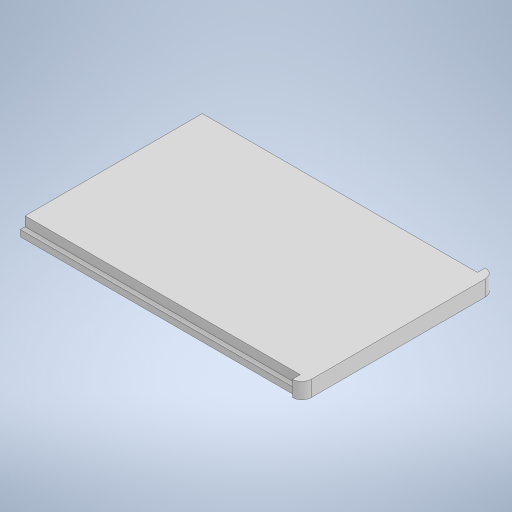
# Autodesk Inventor part: bt-lid
Saved by Autodesk Inventor 2024.2 (Build 282272000, 272)
## iProperties
Created: 2025-05-11
Part Number: bt-lid
Material: Типовые
Document SubType Name: Modeling
Designer: nikit
Density: 1 g/cm^3
Appearance: По умолчанию
Author: nikit
Autodesk Inventor part; units mm, degrees
ref_plane "YZ Plane" through (0, 0, 0) normal (1, 0, 0) x (0, 1, 0)
ref_plane "XZ Plane" through (0, 0, 0) normal (0, 1, 0) x (-1, 0, 0)
ref_plane "XY Plane" through (0, 0, 0) normal (0, 0, 1) x (1, 0, 0)
sketch "Эскиз1" plane through (0, 0, 0) normal (0, 1, 0) x (-1, 0, 0)
  line L0 (43.5, -29.5) -> (-43.5, -29.5)
  line L1 (-43.5, -29.5) -> (-43.5, 29.5)
  line L2 (-43.5, 29.5) -> (43.5, 29.5)
  line L3 (43.5, 29.5) -> (43.5, -29.5)
  line L4 (43.5, -29.5) -> (-43.5, 29.5) construction
  line L5 (-43.5, -29.5) -> (43.5, 29.5) construction
  point P0 (0, 0)
  dimension "d0" = 87
  dimension "d1" = 59
  constraints: 12 end point, 2 midpoint, 2 parallel, 1 horizontal, 1 perpendicular
  measures "d0" distance of L1.end L2.end
  measures "d1" distance of L0.end L1.end
extrude "Выдавливание1" add sketch "Эскиз1" along normal blind 2
sketch "Эскиз2" plane through (0, 2, 0) normal (0, 1, 0) x (1, 0, 0)
  line L0 (43.5, -28) -> (-43.5, -28)
  line L1 (-43.5, -28) -> (-43.5, 28)
  line L2 (-43.5, 28) -> (43.5, 28)
  line L3 (43.5, 28) -> (43.5, -28)
  line L4 (43.5, -28) -> (-43.5, 28) construction
  line L5 (-43.5, -28) -> (43.5, 28) construction
  point P0 (0, 0)
  dimension "d4" = 87
  dimension "d5" = 56
  constraints: 12 end point, 2 midpoint, 2 parallel, 1 horizontal, 1 perpendicular
  measures "d4" distance of L1.end L2.end
  measures "d5" distance of L0.end L1.end
extrude "Выдавливание2" add sketch "Эскиз2" along normal blind 3
sketch "Эскиз3" plane through (0, 0, 0) normal (0, -1, 0) x (1, 0, 0)
  line L0 (43.5, 29.5) -> (43.5, -29.5) projected
  line L1 (43.5, 0) -> (43.5, -30.5)
  line L2 (43.5, 0) -> (43.5, 30.5)
  line L3 (43.5, -30.5) -> (43.5, -27.5)
  circle A0 centre (43.5, -27.5) radius 3
  line L4 (43.5, 0) -> (-8.3438, 0)
  circle A1 centre (43.5, 27.5) radius 3
  line L5 (46.5, 27.5) -> (46.5, -27.5)
  point P0 (0, 0)
  dimension "d8" = 30.5
  dimension "d9" = 30.5
  dimension "d10" = 3
  constraints: 10 end point, 2 point on circle, 2 point on line, 2 vertical, 1 centre point, 1 coincident, 1 collinear, 1 horizontal, 1 midpoint, 1 symmetric about line, 4 other
  measures "d8" distance of L1.start L1.end
  measures "d9" distance of L1.start L2.end
  measures "d10" distance of L1.end L3.end
extrude "Выдавливание3" add sketch "Эскиз3" against normal blind 5 contours L0 A0 L1 | L0 A1 L5 A0 | L0 L2 A1 picked at (44.2818, -28.7902) picked at (43.7225, 26.1917)
